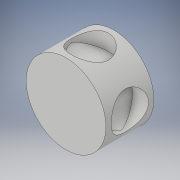
# Autodesk Inventor part: roue
Saved by Autodesk Inventor 2019 (Build 230136000, 136)
## iProperties
Created: 2020-12-11
Part Number: roue
Material: Générique
Document SubType Name: Modeling
Designer: tom.mousset
Density: 1 g/cm^3
Appearance: Par défaut
Author: tom.mousset
Autodesk Inventor part; units mm, degrees
ref_plane "YZ Plane" through (0, 0, 0) normal (1, 0, 0) x (0, 1, 0)
ref_plane "XZ Plane" through (0, 0, 0) normal (0, 1, 0) x (-1, 0, 0)
ref_plane "XY Plane" through (0, 0, 0) normal (0, 0, 1) x (1, 0, 0)
sketch "Esquisse1" plane through (0, 0, 0) normal (0, 0, 1) x (1, 0, 0)
  circle A0 centre (0, 0) radius 15
  ellipse E0 centre (12, 0) end of major axis (12, 7) minor radius 3
  line L0 (12, 7) -> (13.2665, 7)
  line L1 (12, -7) -> (13.2665, -7)
  arc A1 (13.2665, -7) -> (13.2665, 7) centre (0, 0) ccw
  point P0 (15, 0)
  dimension "d2" = 7
  dimension "d3" = 3
  dimension "d0" = 30
  dimension "d1" = 3
  constraints: 6 point on circle, 4 end point, 3 horizontal, 2 centre point, 2 coincident, 1 parallel, 4 other
  measures "d0" diameter of A0
  measures "d1" distance of point (12, 0) A0.start
sketch "Esquisse2" plane through (0, 0, 0) normal (0, 0, 1) x (1, 0, 0)
  circle A0 centre (0, 0) radius 15
  dimension "d4" = 30
  constraints: 1 centre point, 1 coincident
  measures "d4" diameter of A0
extrude "Extrusion1" add sketch "Esquisse2" along normal mid plane 18
sketch "Esquisse3" plane through (0, 0, 0) normal (1, 0, 0) x (0, 1, 0)
  circle A0 centre (0, 0) radius 7
  line L0 (15, 9) -> (-15, 9) projected
  line L1 (-15, -9) -> (15, -9) projected
  line L2 (7.9857, 9) -> (-7.2837, 9)
  line L3 (-7.2837, 9) -> (-7.2837, -9)
  line L4 (-7.2837, -9) -> (7.9857, -9)
  line L5 (7.9857, -9) -> (7.9857, 9)
  dimension "d7" = 14
  constraints: 8 end point, 2 parallel, 2 point on line, 1 centre point, 1 coincident, 1 horizontal, 1 perpendicular
  measures "d7" diameter of A0
extrude "Extrusion2" cut sketch "Esquisse1" along normal mid plane 14 contours A0 E0 L0 | L1 E0 A0 | E0 A0 | A0 E0 | A0 E0
extrude "Extrusion3" add sketch "Esquisse3" along normal blind 16
sketch "Esquisse4" plane through (0, 0, 9) normal (0, 0, 1) x (1, 0, 0)
  circle A0 centre (0, 0) radius 15
  line L0 (-28.9217, 20.5999) -> (24.6243, 20.5999)
  line L1 (24.6243, 20.5999) -> (24.6243, -19.986)
  line L2 (24.6243, -19.986) -> (-28.9217, -19.986)
  line L3 (-28.9217, -19.986) -> (-28.9217, 20.5999)
  constraints: 8 end point, 2 parallel, 1 centre point, 1 coincident, 1 horizontal, 1 perpendicular
extrude "Extrusion4" cut sketch "Esquisse4" against normal blind 18
pattern_circular "Réseau circulaire1" count 4 over 360 about axis through (0, 0, -10) along (0, 0, 1) of "Extrusion2", "Extrusion3", "Extrusion4"
sketch "Esquisse5" plane through (0, 0, -9) normal (0, 0, -1) x (-1, 0, 0)
  circle A0 centre (0, 0) radius 2.6
  line L0 (-1.55, 2.0875) -> (-1.55, -2.0875)
  line L1 (1.55, 2.0875) -> (1.55, -2.0875)
  arc A1 (1.55, 2.0875) -> (-1.55, 2.0875) centre (0, 0) ccw
  arc A2 (-1.55, -2.0875) -> (1.55, -2.0875) centre (0, 0) ccw
  dimension "d25" = 5.2
  dimension "d26" = 1.55
  dimension "d27" = 1.55
  constraints: 8 point on circle, 4 end point, 3 centre point, 3 coincident, 1 parallel, 1 vertical
  measures "d25" diameter of A0
  measures "d26" distance from line of L0 point (0, 0)
  measures "d27" distance from line of point (0, 0) L1
extrude "Extrusion5" cut sketch "Esquisse5" against normal blind 6.2 contours L1 A0 L0
fillet "Congé1" radius 0.5 4 edges at (0, 2.6, -9) (-1.55, 0, -9) (1.55, 0, -9) (0, -2.6, -9)
